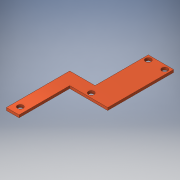
# Autodesk Inventor part: CU3
Saved by Autodesk Inventor 2016 (Build 200138000, 138)
## iProperties
Created: 2018-04-30
Part Number: CU3
Material: Copper
Document SubType Name: Modeling
Designer: Phil Erle
Density: 8.94 g/cm^3
Appearance: Copper - Satin
Author: Phil Erle
Autodesk Inventor part; units mm, degrees
ref_plane "YZ Plane" through (0, 0, 0) normal (1, 0, 0) x (0, 1, 0)
ref_plane "XZ Plane" through (0, 0, 0) normal (0, 1, 0) x (-1, 0, 0)
ref_plane "XY Plane" through (0, 0, 0) normal (0, 0, 1) x (1, 0, 0)
sketch "Sketch1" plane through (0, 0, 0) normal (0, 0, 1) x (1, 0, 0)
  line L0 (10, 42) -> (-10, 42)
  line L1 (-10, 42) -> (-10, 0)
  line L2 (-10, 0) -> (-30, 0)
  line L3 (-30, 0) -> (-30, -50)
  line L4 (-30, -50) -> (-20, -50)
  line L5 (-20, -50) -> (-20, -10)
  line L6 (-20, -10) -> (10, -10)
  line L7 (10, -10) -> (10, 42)
  point P0 (0, 0)
  point P1 (0, 42)
  dimension "d0" = 10
  dimension "d1" = 10
  dimension "d2" = 20
  dimension "d3" = 52
  dimension "d4" = 50
  dimension "d5" = 30
  constraints: 16 end point, 7 perpendicular, 1 horizontal, 1 horizontal alignment, 1 midpoint, 1 vertical alignment
  measures "d0" distance of L3.end L4.end
  measures "d1" distance between parallel lines of L2 L6
  measures "d2" distance of L0.start L0.end
  measures "d3" distance of L6.end L0.start
  measures "d4" distance of L2.end L3.end
  measures "d5" distance between parallel lines of L7 L5
extrude "Extrusion1" add sketch "Sketch1" along normal blind 2
sketch "Sketch2" plane through (0, 0, 2) normal (0, 0, 1) x (1, 0, 0)
  line L0 (6.5, 38.5) -> (-6.5, 38.5) construction
  line L1 (-6.5, 38.5) -> (-6.5, -6.5) construction
  line L2 (10, 42) -> (-10, 42) projected
  line L3 (-30, -50) -> (-20, -50) projected
  line L4 (-20, -50) -> (-20, -10) projected
  point P0 (0, 0)
  point P1 (0, 38.5)
  point P2 (-25, -44)
  dimension "d8" = 13
  dimension "d9" = 45
  dimension "d10" = 3.5
  dimension "d11" = 10
  dimension "d12" = 5
  dimension "d13" = 37.5
  constraints: 4 end point, 3 coincident, 1 horizontal, 1 midpoint, 1 perpendicular, 1 vertical alignment
  measures "d8" distance of L0.start L0.end
  measures "d9" distance of L0.end L1.end
  measures "d10" distance from line of point (0, 38.5) L2
  measures "d11" distance of L3.start L3.end
  measures "d12" distance from line of L4 point (-25, -44)
  measures "d13" vertical distance of L1.end point (-25, -44)
hole "Hole1" at (-25, -44, 2) at (-6.5, -6.5, 2) at (-6.5, 38.5, 2) at (6.5, 38.5, 2) direction (0, 0, -1) diameter 4.5 depth 8 tip angle 118 clearance for "Countersunk Flat Head Screw DIN EN ISO 2009" size "M4" standard "DIN"
equation "\"d12\" = 0.5 * d11"
body "Solid1"
